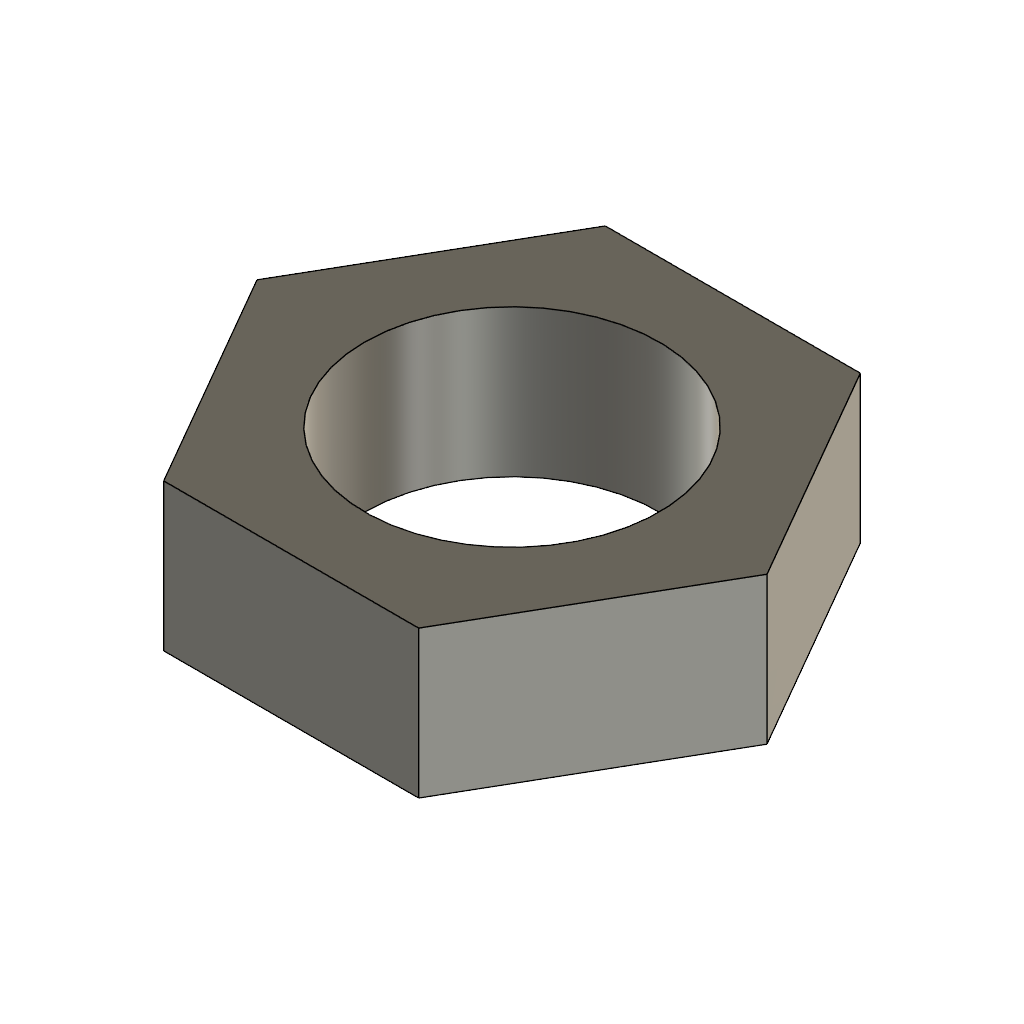
TUERCA_M4 (Autodesk Fusion 360 design; units mm, degrees)
Autodesk Fusion 360 part; units mm, degrees
sketch "Boceto1" plane through (0, 0, 0) normal (0, 0, 1) x (1, 0, 0)
  circle A0 centre (0, 0) radius 2
  line L0 (-1.7321, 3) -> (-3.4641, 0)
  line L1 (-3.4641, 0) -> (-1.7321, -3)
  line L2 (-1.7321, -3) -> (1.7321, -3)
  line L3 (1.7321, -3) -> (3.4641, 0)
  line L4 (3.4641, 0) -> (1.7321, 3)
  line L5 (1.7321, 3) -> (-1.7321, 3)
  dimension "d1" = 4
  constraint coincident A0.centre origin
  measures "d1" diameter of A0
extrude "Extruir1" add sketch "Boceto1" along normal blind 2
